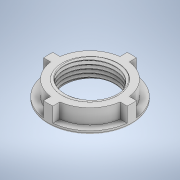
# Autodesk Inventor part: Connector Female
Saved by Autodesk Inventor 2020.2 (Build 242310000, 310)
## iProperties
Created: 2020-04-22
Part Number: Connector Female
Material: Generic
Document SubType Name: Modeling
Designer: a
Density: 1 g/cm^3
Appearance: Default
Author: a
Autodesk Inventor part; units mm, degrees
ref_plane "YZ Plane" through (0, 0, 0) normal (1, 0, 0) x (0, 1, 0)
ref_plane "XZ Plane" through (0, 0, 0) normal (0, 1, 0) x (-1, 0, 0)
ref_plane "XY Plane" through (0, 0, 0) normal (0, 0, 1) x (1, 0, 0)
sketch "Sketch1" plane through (0, 0, 0) normal (0, 1, 0) x (-1, 0, 0)
  circle A0 centre (0, 0) radius 22.5
  circle A1 centre (0, 0) radius 15
  dimension "d0" = 45
  dimension "d1" = 30
  constraints: 2 centre point, 2 coincident
  measures "d0" diameter of A0
  measures "d1" diameter of A1
extrude "Washer" add sketch "Sketch1" along normal blind 2
sketch "Sketch2" plane through (0, 2, 0) normal (0, 1, 0) x (1, 0, 0)
  circle A0 centre (0, 0) radius 18.75
  circle A1 centre (0, 0) radius 15
  circle A2 centre (0, 0) radius 15 projected
  line L0 (-18.5826, -2.5) -> (-22.3607, -2.5)
  circle A3 centre (0, 0) radius 22.5 projected
  line L1 (-18.5826, 2.5) -> (-22.3607, 2.5)
  arc A4 (-22.3607, 2.5) -> (-22.3607, -2.5) centre (0, 0) ccw
  line L2 (-31.5, 0) -> (31.5, 0) projected
  line L3 (-2.5, -18.5826) -> (-2.5, -22.3607)
  arc A5 (-2.5, -22.3607) -> (2.5, -22.3607) centre (0, 0) ccw
  line L4 (2.5, -18.5826) -> (2.5, -22.3607)
  line L5 (18.5826, -2.5) -> (22.3607, -2.5)
  arc A6 (22.3607, -2.5) -> (22.3607, 2.5) centre (0, 0) ccw
  line L6 (18.5826, 2.5) -> (22.3607, 2.5)
  line L7 (2.5, 18.5826) -> (2.5, 22.3607)
  arc A7 (2.5, 22.3607) -> (-2.5, 22.3607) centre (0, 0) ccw
  line L8 (-2.5, 18.5826) -> (-2.5, 22.3607)
  point P0 (2.5, 18.5826)
  point P1 (18.5826, -2.5)
  point P2 (-2.5, -18.5826)
  dimension "d9" = 5
  dimension "d12" = 360
  dimension "d115" = 37.5
  constraints: 16 end point, 12 point on circle, 6 centre point, 2 coincident, 2 concentric, 1 horizontal, 1 parallel, 34 other
  measures "d9" distance between parallel lines of L1 L0
  measures "d115" diameter of A0
extrude "Nut" add sketch "Sketch2" along normal blind 8 contours L2 A1 A0 | L2 A3 L5 A0 | A0 L2 A1 | A0 L6 A3 L2 | A0 L8 A3 L7 | L4 A3 L3 A0 | L2 A3 L1 A0 | A0 L0 A3 L2
fillet "Fillet1" radius 1 1 edges at (22.5, 0, 0)
thread "Thread8" size "M30x2" class "6H" standard "ANSI Metric M Profile" full length
sketch "Sketch16" plane through (0, 10, 0) normal (1, 0, 0) x (0, 0, 1)
  line L0 (15, 0) -> (15, 10)
  line L1 (15, 10) -> (13.5171, 10)
  line L2 (13.5171, 10) -> (13.5171, 0)
  line L3 (13.5171, 0) -> (15, 0)
  line L4 (0, -4.6171) -> (0, 12.4362) projected
  constraints: 8 end point
revolve "Revolution7" add sketch "Sketch16" angle 360 about axis through (0, 10, 0) along (0, -1, 0) separate body
sketch "Sketch15" plane through (0, 10, 15) normal (-1, 0, 0) x (0, -1, 0)
  line L0 (-1.1668, -0.1013) -> (-1.0001, -0.1013) construction
  line L1 (0.1666, -1.382) -> (-0.0001, -1.7021) construction
  line L2 (-2.0001, -1.7021) -> (-2.1668, -1.382) construction
  line L3 (-0.8334, -0.1013) -> (-1.0001, 0.2189) construction
  line L4 (-1.0001, 0.2189) -> (-1.1668, -0.1013) construction
  line L5 (-2.0001, -1.7021) -> (-1.8334, -1.382) construction
  line L6 (-0.8334, -0.1013) -> (-0.1668, -1.382)
  line L7 (-2.1668, -1.382) -> (-1.8334, -1.382) construction
  arc A0 (-2.1668, -1.382) -> (-2.0001, -1.4831) centre (-2.0001, -1.2952) ccw construction
  line L8 (0.1666, -1.382) -> (-0.1668, -1.382) construction
  line L9 (-2.0001, -1.7021) -> (-2.0001, -1.382) construction
  line L10 (-0.0001, -1.7021) -> (-0.0001, -1.382) construction
  line L11 (-1.0001, 0.2189) -> (-1.0001, -0.0002) construction
  line L12 (-2.0001, -1.4831) -> (-0.0001, -1.4831)
  arc A1 (-2.0001, -1.4831) -> (-1.8334, -1.382) centre (-2.0001, -1.2952) ccw
  line L13 (-0.1668, -1.382) -> (-0.0001, -1.7021) construction
  line L14 (-1.8334, -1.382) -> (-1.1668, -0.1013)
  line L15 (-0.0001, -0.0002) -> (-0.0001, 0.0177)
  line L16 (-0.0001, 0.0177) -> (-0.0001, -0.0002)
  line L17 (-0.0001, -0.0002) -> (0.0334, -0.0002)
  arc A2 (-0.1668, -1.382) -> (-0.0001, -1.4831) centre (-0.0001, -1.2952) ccw
  arc A3 (-0.0001, -1.4831) -> (0.1666, -1.382) centre (-0.0001, -1.2952) ccw construction
  arc A4 (-1.0001, -0.0002) -> (-1.1668, -0.1013) centre (-1.0001, -0.1881) ccw
  arc A5 (-0.8334, -0.1013) -> (-1.0001, -0.0002) centre (-1.0001, -0.1881) ccw
  line L18 (-1.0001, -0.0002) -> (-1.0001, -0.1013) construction
  line L19 (-1.0001, -0.1013) -> (-0.8334, -0.1013) construction
  dimension "d139" = 55
  dimension "d140" = 0.3202
  dimension "d141" = 0.3202
  dimension "Sketch15_ThreadOffset" = 0
  dimension "Sketch15_MajorRadius" = 1.4829
  dimension "d144" = 2
  dimension "Sketch15_MinorRadius" = 0
  constraints: 40 end point, 12 point on circle, 10 parallel, 8 tangent, 6 centre point, 6 collinear, 2 midpoint, 2 point on line, 1 horizontal, 1 perpendicular, 3 other
  measures "d139" angle of L6 L14
  measures "d140" distance of L3.end L0.end
  measures "d141" distance of L1.end L10.end
  measures "Sketch15_ThreadOffset" distance between parallel lines of L15 L10
  measures "Sketch15_MajorRadius" distance from line of L12 L15.start
  measures "d144" distance from line of L1.end L9
  measures "Sketch15_MinorRadius" distance edge to line of A5 L17
coil "Coil7" sketch "Sketch15" operation cut axis through (0, 10, 0) along (0, -1, 0) pitch 2.002 turns 6.993007 hand right bodies 2
equation "\"d0\" = Washer_D"
equation "\"d1\" = Thread_D"
equation "\"d2\" = Washer_T"
equation "\"d115\" = 0.5 * Washer_D + 0.5 * Thread_D"
equation "\"d136\" = 0.5 * Washer_T"
equation "\"d139\" = d146"
equation "\"d140\" = 0.160083 * Sketch15_Pitch"
equation "\"d141\" = 0.160083 * Sketch15_Pitch"
equation "\"d144\" = Sketch15_Pitch"
equation "\"d23\" = 55deg"
equation "\"Sketch3_Pitch\" = 1"
equation "\"d43\" = 55deg"
equation "\"Sketch5_Pitch\" = 1"
equation "\"d63\" = 55deg"
equation "\"Sketch7_Pitch\" = 1"
equation "\"d83\" = 55deg"
equation "\"Sketch9_Pitch\" = 1"
equation "\"d104\" = 55deg"
equation "\"Sketch11_Pitch\" = 2"
equation "\"Thread_D\" = 30"
equation "\"Washer_D\" = 45"
equation "\"d125\" = 55deg"
equation "\"Sketch13_Pitch\" = 2"
equation "\"Washer_T\" = 2"
equation "\"d146\" = 55deg"
equation "\"Sketch15_Pitch\" = 2"
body "Solid1"
body "Solid8"
